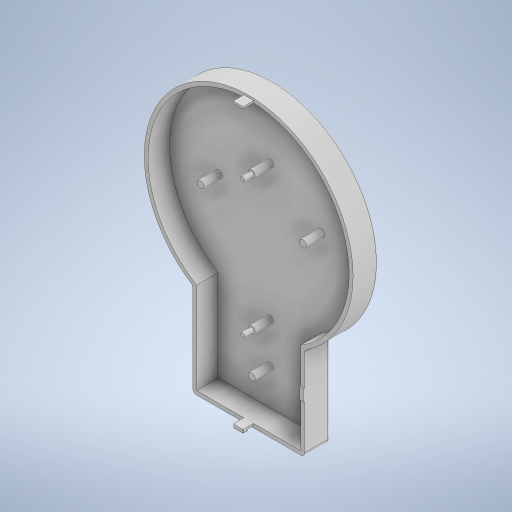
# Autodesk Inventor part: BottomBox
Saved by Autodesk Inventor 2024 (Build 280153000, 153)
## iProperties
Created: 2023-11-16
Part Number: BottomBox
Material: Générique
Document SubType Name: Modeling
Designer: digiacom
Density: 1 g/cm^3
Appearance: Par défaut
Author: digiacom
Autodesk Inventor part; units mm, degrees
ref_plane "YZ Plane" through (0, 0, 0) normal (1, 0, 0) x (0, 1, 0)
ref_plane "XZ Plane" through (0, 0, 0) normal (0, 1, 0) x (-1, 0, 0)
ref_plane "XY Plane" through (0, 0, 0) normal (0, 0, 1) x (1, 0, 0)
sketch "Esquisse1" plane through (0, 0, 0) normal (0, 0, 1) x (1, 0, 0)
  circle A0 centre (0, 0) radius 51
  line L0 (0, 0) -> (-26.4, 0)
  line L1 (-26.4, 0) -> (-26.4, -90)
  line L2 (-26.4, -90) -> (0, -90)
  line L3 (0, -90) -> (0, 0)
  line L4 (0, 0) -> (26.4, 0)
  line L5 (26.4, 0) -> (26.4, -90)
  line L6 (26.4, -90) -> (0, -90)
  line L7 (0, -90) -> (0, 0)
  point P0 (26.4, -43.6353)
  point P1 (-26.4, -43.6353)
  dimension "d5" = 102
  dimension "d6" = 26.4
  dimension "d7" = 90
  dimension "d8" = 26.4
  constraints: 16 end point, 4 parallel, 2 horizontal, 2 perpendicular, 1 centre point, 1 coincident, 1 point on line
  measures "d5" diameter of A0
  measures "d6" distance of L2.end L1.end
  measures "d7" distance of L1.end L0.end
  measures "d8" distance of L5.end L6.end
extrude "Extrusion2" add sketch "Esquisse1" along normal blind 2
sketch "Esquisse2" plane through (0, 0, 2) normal (0, 0, 1) x (1, 0, 0)
  circle A0 centre (0, -50.9) radius 1.75
  line L0 (-26.4, -90) -> (26.4, -90) projected
  line L1 (-26.4, -43.6353) -> (-26.4, -90) projected
  circle A1 centre (0, 17.68) radius 1.75
  point P0 (0, 0)
  dimension "d11" = 3.5
  dimension "d12" = 39.1
  dimension "d13" = 26.4
  dimension "d19" = 3.5
  dimension "d20" = 107.68
  dimension "d21" = 26.4
  constraints: 2 centre point
  measures "d11" diameter of A0
  measures "d12" distance from line of L0 A0.centre
  measures "d13" distance from line of L1 A0.centre
  measures "d19" diameter of A1
  measures "d20" distance from line of L0 A1.centre
  measures "d21" distance from line of L1 A1.centre
extrude "Extrusion5" add sketch "Esquisse2" along normal blind 9.2
sketch "Esquisse4" plane through (0, -50.9, 11.2) normal (0, 0, 1) x (1, 0, 0)
  circle A0 centre (0, 0) radius 1
  point P0 (0, 50.9)
  dimension "d24" = 2
  constraints: 1 centre point
  measures "d24" diameter of A0
sketch "Esquisse5" plane through (0, 17.68, 11.2) normal (0, 0, 1) x (1, 0, 0)
  circle A0 centre (0, 0) radius 1.75 projected
  circle A1 centre (0, 0) radius 1
  point P0 (0, -17.68)
  dimension "d25" = 2
  constraints: 1 centre point, 1 coincident
  measures "d25" diameter of A1
extrude "Extrusion6" add sketch "Esquisse4" along normal blind 4.6
extrude "Extrusion7" add sketch "Esquisse5" along normal blind 4.6 contours A1
sketch "Esquisse6" plane through (0, 0, 2) normal (0, 0, 1) x (1, 0, 0)
  circle A0 centre (0, -71.5) radius 1.75
  line L0 (-26.4, -90) -> (26.4, -90) projected
  circle A1 centre (26, 0) radius 1.75
  circle A2 centre (-26, 0) radius 1.75
  point P0 (0, 0)
  dimension "d30" = 3.5
  dimension "d31" = 18.5
  dimension "d32" = 3.5
  dimension "d33" = 3.5
  dimension "d34" = 26
  dimension "d37" = 26
  constraints: 3 centre point
  measures "d30" diameter of A0
  measures "d31" distance from line of L0 A0.centre
  measures "d32" diameter of A1
  measures "d33" diameter of A2
  measures "d34" distance of point (0, 0) A1.centre
  measures "d37" distance of point (0, 0) A2.centre
extrude "Extrusion8" add sketch "Esquisse6" along normal blind 9.2
sketch "Esquisse7" plane through (0, 0, 0) normal (0, 0, -1) x (-1, 0, 0)
  circle A0 centre (0, 0) radius 53
  line L0 (-28.4, -92) -> (28.4, -92)
  line L1 (28.4, -92) -> (28.4, -31.2211)
  line L2 (28.4, -31.2211) -> (-28.4, -31.2211)
  line L3 (-28.4, -31.2211) -> (-28.4, -92)
  line L4 (26.4, -43.6353) -> (26.4, -90) projected
  line L5 (26.4, -90) -> (-26.4, -90) projected
  line L6 (-26.4, -90) -> (-26.4, -43.6353) projected
  circle A1 centre (0, 0) radius 51
  line L7 (-26.4, -90) -> (26.4, -90)
  line L8 (26.4, -90) -> (26.4, -31.2211)
  line L9 (26.4, -31.2211) -> (-26.4, -31.2211)
  line L10 (-26.4, -31.2211) -> (-26.4, -90)
  point P0 (-26.4, -66.8177)
  point P1 (28.4, -44.7486)
  point P2 (-28.4, -44.7486)
  dimension "d38" = 106
  dimension "d39" = 2
  dimension "d40" = 2
  dimension "d41" = 60.7789
  dimension "d42" = 2
  constraints: 16 end point, 4 parallel, 2 centre point, 2 coincident, 2 horizontal, 2 perpendicular, 1 midpoint, 1 point on line
  measures "d38" diameter of A0
  measures "d39" distance between parallel lines of L4 L1
  measures "d40" distance between parallel lines of L5 L0
  measures "d41" distance of L2.end L0.start
  measures "d42" distance from line of L3 point (-26.4, -66.818)
extrude "Extrusion10" add sketch "Esquisse7" against normal blind 12.8 contours A0 L1 A1 L3 | L3 A1 L6 A0 | A0 L6 L5 L4 L1 L0 L3 | A0 L4 A1 L1
fillet "Congé2" radius 1 4 edges at (0, 53, 0) (-28.4, -68.3743, 0) (0, -92, 0) (28.4, -68.3743, 0)
fillet "Congé3" radius 2 8 edges at (28.1071, -91.7071, 0.2929) (28.4, -92, 6.9) (-28.1071, -91.7071, 0.2929) (-28.4, -92, 6.9) (-28.0904, -44.5781, 0.2766) (-28.4, -44.7486, 6.9) (28.0904, -44.5781, 0.2766) (28.4, -44.7486, 6.9)
sketch "Esquisse8" plane through (28.4, -90, 12.8) normal (1, 0, 0) x (0, 0, -1)
  line L0 (0, 0) -> (0, 44.1651) projected
  line L1 (0, 22.55) -> (-0.5, 22.55)
  line L2 (-0.5, 22.55) -> (-0.5, 28.45)
  line L3 (-0.5, 28.45) -> (0, 28.45)
  line L4 (0, 28.45) -> (0, 22.55)
  line L5 (11.8, 0) -> (0, 0) projected
  point P0 (12.8, 90)
  point P1 (-0.25, 22.55)
  point P2 (-0.25, 28.45)
  point P3 (0, 28.45)
  dimension "d50" = 5.9
  dimension "d51" = 0.5
  dimension "d52" = 28.45
  constraints: 8 end point, 2 midpoint, 2 parallel, 1 horizontal, 1 perpendicular, 1 point on line
  measures "d50" distance of point (-0.25, 22.55) point (-0.25, 28.45)
  measures "d51" distance between parallel lines of L0 L2
  measures "d52" distance between parallel lines of L5 L3
extrude "Extrusion11" add sketch "Esquisse8" against normal blind 2
sketch "Esquisse9" plane through (0, 0, 12.8) normal (0, 0, 1) x (1, 0, 0)
  line L0 (26.4, -90) -> (-26.4, -90) projected
  line L1 (-2.5, -90) -> (2.5, -90)
  line L2 (2.5, -90) -> (2.5, -91)
  line L3 (2.5, -91) -> (-2.5, -91)
  line L4 (-2.5, -91) -> (-2.5, -90)
  line L5 (28.4, -90) -> (28.4, -67.45) projected
  line L6 (-28.4, -45.8349) -> (-28.4, -90) projected
  point P0 (0, 0)
  point P1 (-2.5, -90.5)
  dimension "d55" = 5
  dimension "d56" = 1
  dimension "d57" = 25.9
  dimension "d58" = 25.9
  constraints: 8 end point, 2 parallel, 1 horizontal, 1 midpoint, 1 perpendicular, 1 point on line
  measures "d55" distance of L2.end L3.end
  measures "d56" distance of L1.end L2.end
  measures "d57" distance between parallel lines of L5 L2
  measures "d58" distance from line of L6 point (-2.5, -90.5)
extrude "Extrusion12" add sketch "Esquisse9" along normal blind 5.378
sketch "Esquisse10" plane through (-2.5, -91, 12.8) normal (0, -1, 0) x (1, 0, 0)
  line L0 (5, 5.378) -> (0, 5.378) projected
  line L1 (5, 0) -> (5, 5.378) projected
  line L2 (0, 5.378) -> (5, 5.378)
  line L3 (5, 5.378) -> (5, 2.878)
  line L4 (5, 2.878) -> (0, 2.878)
  line L5 (0, 2.878) -> (0, 5.378)
  point P0 (2.5, -12.8)
  dimension "d61" = 2.5
  constraints: 8 end point, 2 parallel, 1 horizontal, 1 perpendicular, 1 point on line
  measures "d61" distance of L2.end L3.end
extrude "Extrusion13" add sketch "Esquisse10" along normal blind 1
fillet "Congé4" radius 0.5 1 edges at (0, -92, 15.678)
fillet "Congé6" radius 0.4 9 edges at (0, -92, 18.178) (2.5, -91.8536, 15.8244) (2.5, -91.25, 15.678) (2.5, -92, 17.178) (-2.5, -91.8536, 15.8244) (-2.5, -91.25, 15.678) (-2.5, -92, 17.178) (2.5, -91, 18.178) (-2.5, -91, 18.178)
sketch "Esquisse11" plane through (0, 0, 12.8) normal (0, 0, 1) x (1, 0, 0)
  arc A0 (26.4, -43.6353) -> (-26.4, -43.6353) centre (0, 0) ccw projected
  arc A1 (0, 51) -> (-2.4992, 50.9387) centre (0, 0) ccw
  arc A2 (2.4992, 50.9387) -> (0, 51) centre (0, 0) ccw
  line L0 (-2.4992, 50.9387) -> (-2.5483, 51.9375)
  arc A3 (27.4, -44.1955) -> (-27.4, -44.1955) centre (0, 0) ccw projected
  line L1 (2.4992, 50.9387) -> (2.5483, 51.9375)
  arc A4 (2.5483, 51.9375) -> (-2.5483, 51.9375) centre (0, 0) ccw
  dimension "d67" = 2.5
  dimension "d68" = 2.5
  dimension "d69" = 1
  dimension "d70" = 1
  constraints: 11 point on circle, 4 end point, 3 centre point, 2 concentric
  measures "d67" distance of A1.start L0.start
  measures "d68" distance of A1.start L1.start
  measures "d69" distance of L0.start L0.end
  measures "d70" distance of L1.start L1.end
extrude "Extrusion14" add sketch "Esquisse11" along normal blind 5.378
equation "\"d21\" = d13"
equation "\"d34\" = d37"
